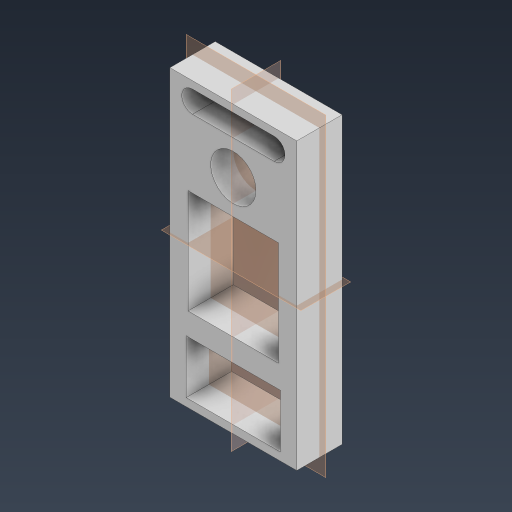
# Autodesk Inventor part: Крепление_TCRT
Saved by Autodesk Inventor 2023.2 (Build 272271030, 271C)
## iProperties
Created: 2025-12-27
Part Number: Крепление_TCRT
Material: Типовые
Document SubType Name: Modeling
Designer: Олег Коноваленко
Density: 1 g/cm^3
Appearance: По умолчанию
Author: Олег Коноваленко
Autodesk Inventor part; units mm, degrees
sketch "Эскиз1" plane through (0, 0, 0) normal (0, 0, 1) x (1, 0, 0)
  line L0 (-7, -15.75) -> (7, -15.75)
  line L1 (7, -15.75) -> (7, 15.75)
  line L2 (7, 15.75) -> (-7, 15.75)
  line L3 (-7, 15.75) -> (-7, -15.75)
  line L4 (-7, -15.75) -> (7, 15.75) construction
  line L5 (7, -15.75) -> (-7, 15.75) construction
  point P0 (0, 0)
  dimension "d0" = 14
  dimension "d1" = 31.5
  constraints: 12 end point, 2 midpoint, 2 parallel, 1 horizontal, 1 perpendicular
  measures "d0" distance of L1.end L2.end
  measures "d1" distance of L0.end L1.end
extrude "Выдавливание1" add sketch "Эскиз1" along normal mid plane 5
sketch "Эскиз2" plane through (0, 0, -2.5) normal (0, 0, -1) x (-1, 0, 0)
  circle A0 centre (0, 8.75) radius 1.5 projected
  circle A1 centre (0, 8.75) radius 2.5
  point P0 (0, 0)
  dimension "d7" = 1
  constraints: 1 centre point
  measures "d7" radial gap between concentric circles of A0 A1
sketch "Эскиз3" plane through (0, 0, -2.5) normal (0, 0, -1) x (-1, 0, 0)
  line L0 (-5.2, -14.88) -> (5.2, -14.88)
  line L1 (5.2, -14.88) -> (5.2, -8.98)
  line L2 (5.2, -8.98) -> (-5.2, -8.98)
  line L3 (-5.2, -8.98) -> (-5.2, -14.88)
  line L4 (-5.2, -14.88) -> (5.2, -8.98) construction
  line L5 (5.2, -14.88) -> (-5.2, -8.98) construction
  line L6 (-7, -15.75) -> (7, -15.75) projected
  line L7 (0, -22.05) -> (0, 22.05) construction
  point P0 (0, 0)
  point P1 (0, -11.93)
  dimension "d4" = 0.87
  dimension "d5" = 5.9
  dimension "d6" = 10.4
  constraints: 12 end point, 2 midpoint, 2 parallel, 1 horizontal, 1 perpendicular, 1 point on line
  measures "d4" distance between parallel lines of L6 L0
  measures "d5" distance of L2.end L0.start
  measures "d6" distance of L1.end L2.end
extrude "Выдавливание2" cut sketch "Эскиз2" against normal up to next contours A0 | A1
extrude "Выдавливание3" cut sketch "Эскиз3" against normal up to next
sketch "Эскиз4" plane through (0, 0, 2.5) normal (0, 0, 1) x (1, 0, 0)
  line L0 (-4.5, 13.75) -> (4.5, 13.75) construction
  line L1 (-4.5, 12.55) -> (4.5, 12.55)
  line L2 (4.5, 14.95) -> (-4.5, 14.95)
  arc A0 (-4.5, 14.95) -> (-4.5, 12.55) centre (-4.5, 13.75) ccw
  arc A1 (4.5, 12.55) -> (4.5, 14.95) centre (4.5, 13.75) ccw
  line L3 (7, 15.75) -> (-7, 15.75) projected
  line L4 (0, 22.05) -> (0, -22.05) construction
  point P0 (0, 0)
  point P1 (0, 13.75)
  dimension "d12" = 9
  dimension "d13" = 1.2
  dimension "d14" = 2
  constraints: 8 end point, 4 point on circle, 4 tangent, 2 centre point, 1 horizontal, 1 midpoint, 1 parallel, 1 point on line
  measures "d12" distance of L0.start L0.end
  measures "d13" distance between parallel lines of L2 L0
  measures "d14" distance between parallel lines of L3 L0
extrude "Выдавливание4" cut sketch "Эскиз4" against normal up to next
sketch "Эскиз5" plane through (0, 0, 2.5) normal (0, 0, 1) x (1, 0, 0)
  line L0 (-9.8, 0) -> (9.8, 0) construction
  line L1 (-5, 0) -> (5, 0) construction
  line L2 (5, 0) -> (5, -6.5)
  line L3 (5, -6.5) -> (-5, -6.5)
  line L4 (-5, -6.5) -> (-5, 0)
  line L5 (-5, 0) -> (5, 0) construction
  line L6 (5, 0) -> (5, 5)
  line L7 (5, 5) -> (-5, 5)
  line L8 (-5, 5) -> (-5, 0)
  line L9 (-5, 5) -> (5, -6.5) construction
  line L10 (5, 5) -> (-5, -6.5) construction
  line L11 (0, 22.05) -> (0, -22.05) construction
  point P0 (0, -0.75)
  dimension "d22" = 6.5
  dimension "d23" = 5
  dimension "d24" = 10
  constraints: 20 end point, 4 parallel, 3 point on line, 2 horizontal, 2 perpendicular, 1 midpoint
  measures "d22" distance between parallel lines of L0 L3
  measures "d23" distance between parallel lines of L0 L7
  measures "d24" distance between parallel lines of L6 L8
extrude "Выдавливание5" cut sketch "Эскиз5" against normal up to next
